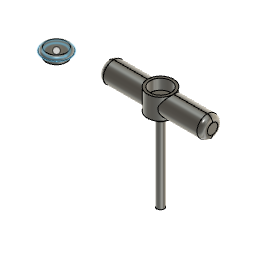
_handle2.e6effeca-72ad-4018-b7d1-6c4084fdfae2 (Autodesk Fusion 360 design; units mm, degrees)
Autodesk Fusion 360 part; units mm, degrees
note: some values were not read from the file. Set by a fixed rule: which sketch regions a step uses.
sketch "Sketch1" plane through (0, 0, 0) normal (0, 0, 1) x (1, 0, 0)
  circle A0 centre (0, 0) radius 2.5
  circle A1 centre (0, 0) radius 3.5
  circle A2 centre (0, 0) radius 10
  circle A3 centre (0, 0) radius 12.5
  line L0 (50, -10) -> (-50, -10)
  line L1 (-50, -10) -> (-50, 10)
  line L2 (-50, 10) -> (50, 10)
  line L3 (50, 10) -> (50, -10)
  line L4 (50, -10) -> (-50, 10) construction
  line L5 (-50, -10) -> (50, 10) construction
  circle A4 centre (0, 0) radius 6
  dimension "d1" = 5
  dimension "d2" = 7
  dimension "d3" = 20
  dimension "d4" = 25
  dimension "d5" = 100
  dimension "d36" = 12
  constraint coincident A0.centre A1.centre
  constraint concentric A0 A1
  constraint concentric A1 A3
  constraint horizontal L0
  constraint perpendicular L0 L1
  constraint parallel L0 L2
  constraint parallel L1 L3
  constraint coincident L4 A0.centre
  constraint coincident L5 A0.centre
  measures "d1" diameter of A0
  measures "d2" diameter of A1
  measures "d3" diameter of A2
  measures "d4" diameter of A3
  measures "d5" distance of L1.end L2.end
  measures "d36" diameter of A4
extrude "Extrude6" add sketch "Sketch1" against normal blind 5 contours A4 makes body 1
extrude "Extrude2" add sketch "Sketch1" along normal blind 10 separate body contours A1 | A2 | A4 makes body 2
extrude "Extrude3" add sketch "Sketch1" along normal blind 20 contours A2 A3 L0 L2 | A2 A3 L0 L2 | A3 L2 | A3 L0 | A3 L0 L1 L2 | A3 L0 L2 L3 bodies 2
extrude "Extrude1" add sketch "Sketch1" against normal blind 80 separate body contours A1 makes body 3
fillet "Fillet1" radius 10 1 edges at (-28.75, -10, 20) on bodies 2
fillet "Fillet2" radius 10 1 edges at (28.75, -10, 20) on bodies 2
fillet "Fillet3" radius 10 1 edges at (28.75, 10, 20) on bodies 2
fillet "Fillet4" radius 10 1 edges at (-28.75, 10, 20) on bodies 2
fillet "Fillet5" radius 10 4 edges at (-28.75, -10, 0) (28.75, -10, 0) (28.75, 10, 0) (-28.75, 10, 0) on bodies 2
fillet "Fillet6" radius 5 2 edges at (50, -10, 10) (50, 10, 10) on bodies 2
fillet "Fillet7" radius 5 2 edges at (-50, -10, 10) (-50, 10, 10) on bodies 2
sketch "Sketch2" plane through (0, 0, 0) normal (0, 0, 1) x (1, 0, 0)
  circle A0 centre (-100, 0) radius 8.5
  circle A1 centre (-100, 0) radius 9.5
  circle A2 centre (-100, 0) radius 12.5
  dimension "d26" = 17
  dimension "d27" = 19
  dimension "d28" = 25
  constraint concentric A0 A1
  constraint concentric A1 A2
  measures "d26" diameter of A0
  measures "d27" diameter of A1
  measures "d28" diameter of A2
extrude "Extrude5" add sketch "Sketch2" along normal blind 3 separate body contours A0 | A1 | A2 makes body 4
extrude "Extrude4" add sketch "Sketch2" against normal blind 5 separate body contours A1 makes body 5
combine "Combine1" operation add target body 4 tool bodies 5
fillet "Fillet8" radius 3 1 edges at (-111.6541, -4.5202, 3) on bodies 4
combine "Combine2" operation add target body 2 tool bodies 1 3
